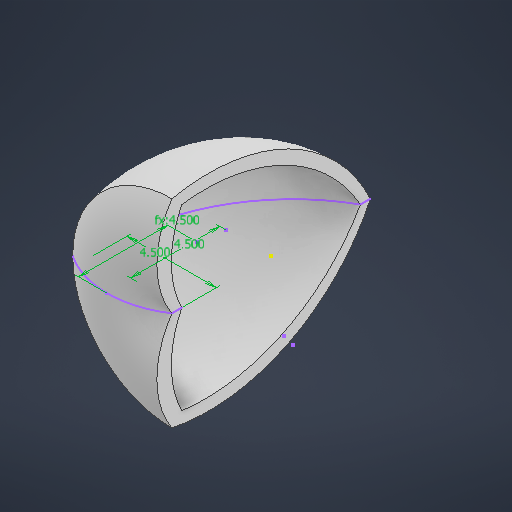
# Autodesk Inventor part: top1
Saved by Autodesk Inventor 2026.1 (Build 301233000, 233)
## iProperties
Created: 2026-04-07
Part Number: top1
Material: Generic
Document SubType Name: Modeling
Designer: Kasi Pusuluri
Density: 1 g/cm^3
Appearance: Default
Author: Kasi Pusuluri
Autodesk Inventor part; units mm, degrees
ref_plane "YZ Plane" through (0, 0, 0) normal (1, 0, 0) x (0, 1, 0)
ref_plane "XZ Plane" through (0, 0, 0) normal (0, 1, 0) x (-1, 0, 0)
ref_plane "XY Plane" through (0, 0, 0) normal (0, 0, 1) x (1, 0, 0)
sketch "Sketch1" plane through (0, 0, 0) normal (1, 0, 0) x (0, 1, 0)
  arc A0 (114.3, 114.3) -> (0, 114.3) centre (57.15, 0) ccw
  arc A1 (0, -114.3) -> (114.3, 114.3) centre (-112.3843, 84.7671) ccw
  arc A2 (127, 127) -> (0, 127) centre (63.5, 31.9619) ccw
  arc A3 (0, -127) -> (127, 127) centre (-96.7416, 80.1208) ccw
  line L0 (0, 114.3) -> (0, 127)
  line L1 (0, -114.3) -> (0, -127)
  line L2 (0, 0) -> (0, 114.3)
  point P0 (57.15, 114.3)
  point P1 (63.5, 146.2619)
  dimension "d1" = 114.3
  dimension "d3" = 114.3
  dimension "d4" = 114.3
  dimension "d5" = 114.3
  dimension "d6" = 228.6
  dimension "d8" = 127
  dimension "d10" = 114.3
  dimension "d11" = 228.6
  constraints: 9 point on circle, 6 end point, 4 centre point, 2 vertical, 1 collinear
  measures "d1" distance of L2.start L0.start
  measures "d3" distance of L2.start L1.start
  measures "d4" distance of L0.start A0.start
  measures "d5" distance of point (57.15, 114.3) A0.centre
  measures "d6" radius of A1
  measures "d8" distance of L2.start L1.end
  measures "d10" distance of A2.centre point (63.5, 146.262)
  measures "d11" radius of A3
sketch "Sketch3" plane through (0, 0, 0) normal (0, 1, 0) x (-1, 0, 0)
  arc A0 (114.2997, 114.3) -> (-0.0003, 114.3) centre (57.1497, 0) ccw
  arc A1 (-0.0002, -114.3) -> (114.2997, 114.3) centre (-112.3846, 84.7671) ccw
  arc A2 (126.9997, 127) -> (-0.0003, 127) centre (63.4997, 31.9619) ccw
  arc A3 (-0.0002, -127) -> (126.9997, 127) centre (-96.7419, 80.1208) ccw
  line L0 (-0.0003, 127) -> (-0.0003, 114.3)
  line L1 (-0.0002, -127) -> (-0.0002, -114.3)
  line L2 (-0.0002, -127) -> (-0.0002, -114.3)
  line L3 (-0.0003, 114.3) -> (-0.0003, 127)
  point P0 (0, 0)
  point P1 (57.1497, 114.3)
  point P2 (63.4997, 146.2619)
  dimension "d0" = 114.3
  dimension "d16" = 114.3
  dimension "d17" = 114.3
  dimension "d22" = 114.3
  constraints: 9 point on circle, 8 end point, 4 centre point, 3 vertical, 1 parallel
  measures "d16" distance of L0.end A0.start
  measures "d17" distance of point (57.15, 114.3) A0.centre
  measures "d22" distance of A2.centre point (63.5, 146.262)
revolve "Revolution1" add sketch "Sketch1" angle 180 about axis through (0, 0, 0) along (0, 0, 1)
equation "\"d1\" = d0"
equation "\"d10\" = d5"
equation "\"d11\" = d6"
equation "\"d22\" = d17"
body "Solid1"
